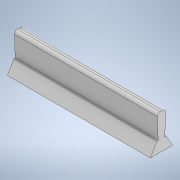
# Autodesk Inventor part: 220525 Notch 0.5 inch
Saved by Autodesk Inventor 2022 (Build 260153000, 153)
## iProperties
Created: 2022-05-25
Part Number: 220525 Notch 0.5 inch
Material: Generic
Document SubType Name: Modeling
Designer: josephinew
Density: 1 g/cm^3
Appearance: Default
Author: josephinew
Autodesk Inventor part; units mm, degrees
ref_plane "YZ Plane" through (0, 0, 0) normal (1, 0, 0) x (0, 1, 0)
ref_plane "XZ Plane" through (0, 0, 0) normal (0, 1, 0) x (-1, 0, 0)
ref_plane "XY Plane" through (0, 0, 0) normal (0, 0, 1) x (1, 0, 0)
sketch "Sketch1" plane through (0, 0, 0) normal (1, 0, 0) x (0, 1, 0)
  arc A0 (63.4973, -0.5882) -> (63.4973, 0.5882) centre (0, 0) ccw
  line L0 (50.7691, -1.7729) -> (61.8544, -2.16)
  line L1 (50.7691, 1.7729) -> (61.8544, 2.16)
  arc A1 (63.4973, 0.5882) -> (61.8544, 2.16) centre (61.9098, 0.5735) ccw
  arc A2 (61.8544, -2.16) -> (63.4973, -0.5882) centre (61.9098, -0.5735) ccw
  arc A3 (2.7261, 50.7268) -> (-2.7261, 50.7268) centre (0, 0) ccw
  line L2 (44.704, 5.9101) -> (44.704, -5.9101)
  line L3 (44.704, 5.9101) -> (50.7421, 2.4239)
  line L4 (44.704, -5.9101) -> (50.7421, -2.4239)
  arc A4 (50.7421, -2.4239) -> (50.7691, -1.7729) centre (0, 0) ccw
  arc A5 (50.7691, 1.7729) -> (50.7421, 2.4239) centre (0, 0) ccw
  line L5 (63.5, 0) -> (73.7693, 0) construction
  point P0 (63.4613, -2.2161)
  point P1 (63.4613, 2.2161)
  point P2 (50.7268, -2.7261)
  dimension "d9" = 1.5875
  constraints: 15 point on circle, 12 end point, 6 centre point, 4 tangent, 2 coincident, 2 point on line, 1 equal radius, 1 horizontal
  measures "d9" radius of A1
extrude "Extrusion1" add sketch "Sketch1" along normal blind 76.2
body "Solid1"
